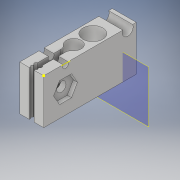
# Autodesk Inventor part: Neuroprobeholdermagiger
Saved by Autodesk Inventor 2017 (Build 210142000, 142)
## iProperties
Created: 2016-08-31
Part Number: Neuroprobeholdermagiger
Material: Generic
Document SubType Name: Modeling
Designer: andrew
Density: 1 g/cm^3
Appearance: Default
Author: andrew
Autodesk Inventor part; units mm, degrees
ref_plane "YZ Plane" through (0, 0, 0) normal (1, 0, 0) x (0, 1, 0)
ref_plane "XZ Plane" through (0, 0, 0) normal (0, 1, 0) x (-1, 0, 0)
ref_plane "XY Plane" through (0, 0, 0) normal (0, 0, 1) x (1, 0, 0)
sketch "Sketch1" plane through (0, 0, 0) normal (0, 1, 0) x (-1, 0, 0)
  line L0 (10.16, 0) -> (10.16, -36.068)
  line L1 (0, -36.068) -> (0, 0) construction
  circle A0 centre (5.08, -25.908) radius 2.9655
  line L2 (10.16, 0) -> (6.096, 0) construction
  line L3 (3.9775, 0) -> (0.0978, 0) construction
  line L4 (4.064, -3.81) -> (4.064, -14.8101) construction
  arc A1 (4.064, -14.8101) -> (6.096, -14.812) centre (5.0772, -17.8191) ccw
  line L5 (5.08, -31.75) -> (24.746, -31.75) construction
  line L6 (0, -4.7834) -> (2.794, -4.7834) construction
  line L7 (2.794, -4.7834) -> (2.794, -13.6734) construction
  line L8 (2.794, -13.6734) -> (0, -13.6734) construction
  line L9 (0, -13.6734) -> (0, -4.7834) construction
  line L10 (4.064, -4.7834) -> (0, -4.7834) construction
  line L11 (5.08, -31.75) -> (9.398, -31.75) construction
  line L12 (10.16, 0) -> (6.096, 0)
  line L13 (4.064, 0) -> (0, 0)
  line L14 (0, 0) -> (0, -36.068)
  line L15 (5.08, -36.068) -> (8.255, -36.068) construction
  line L16 (10.16, -36.068) -> (10.16, -39.243)
  line L17 (10.16, -39.243) -> (0, -39.243)
  line L18 (0, -39.243) -> (0, -36.068)
  line L19 (5.0772, -17.8191) -> (26.8769, -17.8191) construction
  arc A2 (4.064, -0.5428) -> (4.064, -1.7162) centre (4.307, -1.1295) ccw
  line L20 (4.064, -0.5428) -> (4.064, 0)
  arc A3 (4.064, -1.9422) -> (4.064, -3.5201) centre (4.307, -2.7311) ccw
  line L21 (4.064, -14.8101) -> (4.064, -3.5201)
  line L22 (4.064, -1.9422) -> (4.064, -1.7162)
  line L23 (4.064, -3.5201) -> (4.064, -3.81) construction
  line L24 (4.064, 0) -> (4.064, -0.5428) construction
  line L25 (4.064, -1.7162) -> (4.064, -1.9422) construction
  arc A4 (6.0904, -1.7162) -> (6.0904, -0.5428) centre (5.8475, -1.1295) ccw
  arc A5 (6.0904, -3.5201) -> (6.0904, -1.9422) centre (5.8475, -2.7311) ccw
  line L26 (6.096, -0.5451) -> (6.096, 0) construction
  line L27 (6.096, -3.5183) -> (6.096, -14.812)
  line L28 (6.096, 0) -> (6.096, -0.5451)
  line L29 (6.096, -1.7138) -> (6.096, -1.9439)
  line L30 (6.096, -3.81) -> (6.096, -3.5183) construction
  line L31 (6.096, -1.9439) -> (6.096, -1.7138) construction
  dimension "d0" = 10.16
  dimension "d3" = 5.9309
  dimension "d11" = 25.908
  dimension "d18" = 6.35
  dimension "d20" = 8.89
  dimension "d21" = 2.794
  constraints: 64 end point, 14 point on circle, 11 perpendicular, 6 centre point, 6 horizontal, 4 equal length, 3 point on line, 3 vertical
  measures "d0" distance of L0.end L1.start
  measures "d3" diameter of A0
  measures "d11" distance from line of L2 A0.centre
  measures "d18" diameter of A1
  measures "d20" distance of L6.end L7.end
  measures "d21" distance between parallel lines of L9 L7
extrude "Extrusion1" add sketch "Sketch1" along normal blind 19.05
sketch "Sketch2" plane through (0, 0, 0) normal (1, 0, 0) x (0, 0, -1)
  line L0 (39.243, 0) -> (0, 0) construction
  line L1 (0, 19.05) -> (39.243, 19.05) construction
  line L2 (0, 0) -> (0, 19.05) construction
  line L3 (36.068, 9.525) -> (0, 9.525) construction
  line L4 (20.9941, 0) -> (14.812, 0) construction
  line L5 (3.81, 19.05) -> (14.812, 19.05) construction
  line L6 (14.6467, 0) -> (3.81, 0) construction
  line L7 (14.6467, 0) -> (14.6467, 19.05) construction
  line L8 (3.81, 19.05) -> (14.6467, 19.05) construction
  line L9 (3.81, 0) -> (3.81, 19.05) construction
  line L10 (14.6467, 9.525) -> (3.81, 9.525) construction
  circle A0 centre (9.2284, 9.525) radius 1.8542
  line L11 (39.243, 0) -> (39.243, 19.05) projected
  point P0 (14.8101, 0)
  dimension "d26" = 3.7084
  constraints: 4 end point, 4 midpoint, 1 centre point
  measures "d26" diameter of A0
extrude "Extrusion2" cut sketch "Sketch2" against normal blind 19.05
sketch "Sketch3" plane through (0, 19.05, 0) normal (0, 1, 0) x (1, 0, 0)
  line L0 (0, 11.0826) -> (0, 7.3742) projected
  point P0 (0, 0)
sketch "Sketch4" plane through (0, 0, 0) normal (1, 0, 0) x (0, 0, -1)
  circle A0 centre (9.2284, 9.525) radius 1.8542 projected
  line L0 (39.243, 0) -> (0, 0) projected
  line L1 (0, 19.05) -> (39.243, 19.05) projected
  line L2 (0, 0) -> (0, 19.05) projected
  line L3 (14.3084, 9.525) -> (11.7684, 5.1256)
  line L4 (11.7684, 5.1256) -> (6.6884, 5.1256)
  line L5 (6.6884, 5.1256) -> (4.1484, 9.525)
  line L6 (4.1484, 9.525) -> (6.6884, 13.9244)
  line L7 (6.6884, 13.9244) -> (11.7684, 13.9244)
  line L8 (11.7684, 13.9244) -> (14.3084, 9.525)
  line L9 (39.243, 0) -> (39.243, 19.05) projected
  dimension "d30" = 10.16
  constraints: 12 end point, 1 coincident, 13 other
  measures "d30" distance of L5.end L3.start
extrude "Extrusion3" cut sketch "Sketch4" against normal blind 1.778 contours L3 L4 L5 L6 L7 L8
ref_plane "Work Plane1" through (0, 0, -33.528) normal (0, 0, -1) x (-1, 0, 0)
sketch "Sketch6" plane through (0, 0, -33.528) normal (0, 0, -1) x (-1, 0, 0)
  line L0 (0.508, 9.5571) -> (2.8218, 13.5005) projected
  line L1 (7.3938, 13.4684) -> (9.652, 9.4929) projected
  line L2 (2.8218, 13.5005) -> (7.3938, 13.4684) projected
  line L3 (0.508, 9.5571) -> (2.8218, 13.5005) projected
  line L4 (2.7662, 5.5816) -> (0.508, 9.5571) projected
  line L5 (7.3382, 5.5495) -> (2.7662, 5.5816) projected
  line L6 (9.652, 9.4929) -> (7.3382, 5.5495) projected
  circle A0 centre (5.1347, 9.4929) radius 4.5726
  circle A1 centre (5.1347, 9.4929) radius 1.8415
  point P0 (0, 0)
  dimension "d38" = 3.683
  constraints: 1 centre point, 1 coincident, 3 other
  measures "d38" diameter of A1
extrude "Extrusion5" cut sketch "Sketch6" along normal mid plane 12.7 contours A1
sketch "Sketch7" plane through (0, 0, 0) normal (1, 0, 0) x (0, 0, -1)
  line L0 (3.81, 19.05) -> (14.812, 19.05) projected
  circle A0 centre (9.2284, 18.3833) radius 1.27
  line L1 (0, 19.05) -> (39.243, 19.05) projected
  line L2 (6.8407, 19.05) -> (6.8407, 19.558)
  line L3 (6.8407, 19.05) -> (7.3487, 19.05) construction
  line L4 (7.3243, 18.5023) -> (7.3243, 18.3436)
  line L5 (7.3243, 18.5023) -> (7.4831, 18.5023) construction
  line L6 (22.9425, 19.05) -> (28.8734, 19.05) projected
  line L7 (28.8734, 0) -> (22.9425, 0) projected
  line L8 (28.8734, 0) -> (28.8734, 19.05) projected
  line L9 (28.8734, 9.525) -> (35.9855, 9.525)
  line L10 (35.9855, 9.525) -> (32.4294, 9.525)
  circle A1 centre (35.6044, 18.0788) radius 2.286
  line L11 (32.4294, 9.525) -> (32.4294, 7.6962)
  line L12 (32.4294, 7.6962) -> (32.4294, 4.5212)
  line L13 (28.8729, 7.6514) -> (39.243, 7.6514) projected
  line L14 (32.4294, 7.6962) -> (35.6044, 7.6962) construction
  line L15 (32.4294, 4.5212) -> (35.6044, 4.5212)
  point P0 (0, 0)
  point P1 (36.068, 19.05)
  point P2 (28.188, 9.4929)
  dimension "d41" = 2.54
  dimension "d42" = 0.508
  dimension "d43" = 90
  dimension "d46" = 0.1588
  dimension "d47" = 90
  dimension "d48" = 4.572
  dimension "d49" = 1.8288
  dimension "d56" = 3.175
  dimension "d57" = 90
  dimension "d58" = 3.175
  dimension "d59" = 90
  constraints: 20 end point, 6 perpendicular, 4 horizontal, 2 centre point, 2 midpoint, 2 vertical, 1 point on line, 1 other
  measures "d41" diameter of A0
  measures "d42" distance of L2.start L2.end
  measures "d43" angle of L3 L2
  measures "d46" distance of L4.start L4.end
  measures "d47" angle of L4 L5
  measures "d48" diameter of A1
  measures "d49" distance of L10.end L11.end
  measures "d56" distance of L11.end L12.end
  measures "d57" angle of L12 L14
  measures "d58" distance of L12.end L15.end
  measures "d59" angle of L15 L12
extrude "Extrusion6" cut sketch "Sketch7" against normal blind 55.88 contours A0 L0 | A1 L1 | L1 A1 | L0 A0
sketch "Sketch8" plane through (0, 19.05, 0) normal (0, 1, 0) x (1, 0, 0)
  circle A0 centre (-5.08, 25.908) radius 4.191
  point P0 (0, 0)
  dimension "d50" = 8.382
  constraints: 1 centre point, 1 coincident
  measures "d50" diameter of A0
extrude "Extrusion7" cut sketch "Sketch8" against normal blind 6.1214
fillet "Fillet1" radius 2.54 2 edges at (-6.096, 9.525, -14.812) (-4.064, 9.525, -14.8101)
sketch "Sketch9" plane through (-10.16, 0, -39.243) normal (-1, 0, 0) x (0, 0, 1)
  circle A0 centre (30.0146, 9.525) radius 2.0066
  point P0 (39.243, 0)
  dimension "d61" = 4.0132
  constraints: 1 centre point, 1 coincident
  measures "d61" diameter of A0
extrude "Extrusion8" cut sketch "Sketch9" against normal blind 12.7
body "Solid1"
